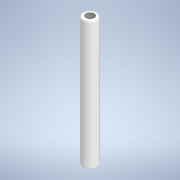
# Autodesk Inventor part: dikey_shaft
Saved by Autodesk Inventor 2020 (Build 240168000, 168)
## iProperties
Created: 2021-12-09
Part Number: dikey_shaft
Material: ABS Plastic
Document SubType Name: Modeling
Designer: Umur Batuhan Özmen
Density: 1.06 g/cm^3
Appearance: Smooth - White
Mass: 23.0343 g
Surface Area: 78.9361 cm^2
Volume: 21.7305 cm^3
Author: Umur Batuhan Özmen
Autodesk Inventor part; units mm, degrees
ref_plane "YZ Plane" through (0, 0, 0) normal (1, 0, 0) x (0, 1, 0)
ref_plane "XZ Plane" through (0, 0, 0) normal (0, 1, 0) x (-1, 0, 0)
ref_plane "XY Plane" through (0, 0, 0) normal (0, 0, 1) x (1, 0, 0)
sketch "Sketch1" plane through (0, 0, 0) normal (0, 1, 0) x (-1, 0, 0)
  circle A0 centre (0, 0) radius 7.5
  dimension "d0" = 15
  constraints: 1 centre point, 1 coincident
  measures "d0" diameter of A0
extrude "Extrusion1" add sketch "Sketch1" along normal blind 137.8
sketch "Sketch2" plane through (0, 137.8, 0) normal (0, 1, 0) x (1, 0, 0)
  circle A0 centre (0, 0) radius 7.5 projected
  circle A1 centre (0, 0) radius 4.4
  dimension "d3" = 8.8
  constraints: 1 centre point, 1 coincident
  measures "d3" diameter of A1
hole "Hole1" at (0, 137.8, 0) direction (0, -1, 0) diameter 9 depth 20
thread "Thread1" size "M9x1.25" class "6H" standard "ISO Metric profile" length 20
sketch "Sketch3" plane through (0, 0, 0) normal (0, -1, 0) x (1, 0, 0)
  circle A0 centre (0, 0) radius 4.4
  dimension "d13" = 8.8
  constraints: 1 centre point, 1 coincident
  measures "d13" diameter of A0
hole "Hole2" at (0, 0, 0) direction (0, 1, 0) diameter 9 depth 20
thread "Thread2" size "M9x1.25" class "6H" standard "ISO Metric profile" length 20
fillet "Fillet1" radius 2 2 edges at (7.5, 137.8, 0) (7.5, 0, 0)
body "Solid1"
